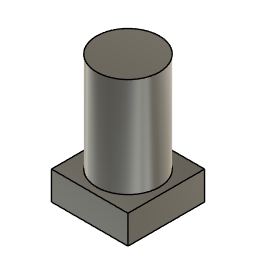
Button+Extension (Autodesk Fusion 360 design; units mm, degrees)
Autodesk Fusion 360 part; units mm, degrees
sketch "Sketch1" plane through (0, 0, 0) normal (0, 0, 1) x (1, 0, 0)
  line L0 (0, 0) -> (10.75, 0)
  line L1 (10.75, 0) -> (10.75, 10.75)
  line L2 (10.75, 10.75) -> (0, 10.75)
  line L3 (0, 10.75) -> (0, 0)
  dimension "d1" = 10.75
  dimension "d2" = 10.75
  constraint horizontal L0
  constraint vertical L1
  constraint horizontal L2
  constraint vertical L3
  constraint coincident L0.start L3.end
  measures "d1" distance of L0.start L0.end
  measures "d2" distance of L0.start L2.end
extrude "Extrude1" add sketch "Sketch1" along normal blind 4
sketch "Sketch2" plane through (0, 0, 4) normal (0, 0, 1) x (-1, 0, 0)
  line L0 (0, -10.75) -> (0, 0)
  line L1 (0, 0) -> (-10.75, 0)
  line L2 (-10.75, 0) -> (-10.75, -10.75)
  line L3 (-10.75, -10.75) -> (0, -10.75)
  circle A0 centre (-5.375, -5.375) radius 4.4
  dimension "d5" = 8.8
  measures "d5" diameter of A0
extrude "Extrude2" add sketch "Sketch2" along normal blind 14 contours A0
